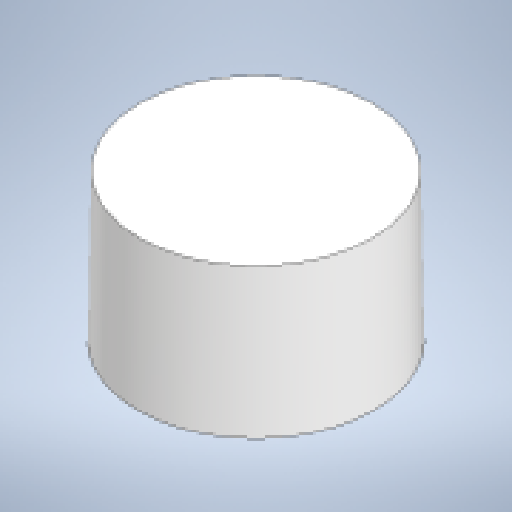
# Autodesk Inventor part: bouchon
Saved by Autodesk Inventor 2024.2 (Build 282272000, 272)
## iProperties
Created: 2024-09-11
Part Number: bouchon
Material: Plastique PPS
Document SubType Name: Modeling
Designer: Sebastien
Density: 1.637 g/cm^3
Appearance: Lisse - Blanc
Author: Sebastien
Autodesk Inventor part; units mm, degrees
ref_plane "YZ Plane" through (0, 0, 0) normal (1, 0, 0) x (0, 1, 0)
ref_plane "XZ Plane" through (0, 0, 0) normal (0, 1, 0) x (-1, 0, 0)
ref_plane "XY Plane" through (0, 0, 0) normal (0, 0, 1) x (1, 0, 0)
sketch "Esquisse1" plane through (0, 0, 0) normal (0, 0, 1) x (1, 0, 0)
  line L0 (28.15, -35) -> (27.6, 0)
  line L1 (27.6, 0) -> (0, 0)
  line L2 (0, 0) -> (0, -3)
  line L3 (0, -3) -> (15.3, -3)
  line L4 (15.3, -3) -> (15.3, -16.6)
  line L5 (15.3, -16.6) -> (16.3, -16.6)
  line L6 (16.3, -16.6) -> (16.3, -1.5)
  line L7 (16.3, -1.5) -> (26.1234, -1.5)
  line L8 (26.1234, -1.5) -> (26.6498, -35)
  line L9 (26.6498, -35) -> (28.15, -35)
  dimension "d0" = 35
  dimension "d1" = 55.2
  dimension "d2" = 56.3
  dimension "d3" = 1.5
  dimension "d4" = 32.6
  dimension "d5" = 1
  dimension "d7" = 18.4
  dimension "d8" = 33.5
  dimension "d10" = 3
  constraints: 20 end point, 6 perpendicular, 1 horizontal, 1 parallel
  measures "d0" distance between parallel lines of L9 L1
  measures "d1" diameter of L0.end L2
  measures "d2" diameter of L0.start L2
  measures "d3" distance between parallel lines of L0 L8
  measures "d4" diameter of L6 L2
  measures "d5" distance of L4.end L5.end
  measures "d7" distance between parallel lines of L9 L5
  measures "d8" distance between parallel lines of L9 L7
  measures "d10" distance between parallel lines of L1 L3
revolve "Révolution1" add sketch "Esquisse1" angle 360 about axis through (0, 0, 0) along (0, -1, 0)
